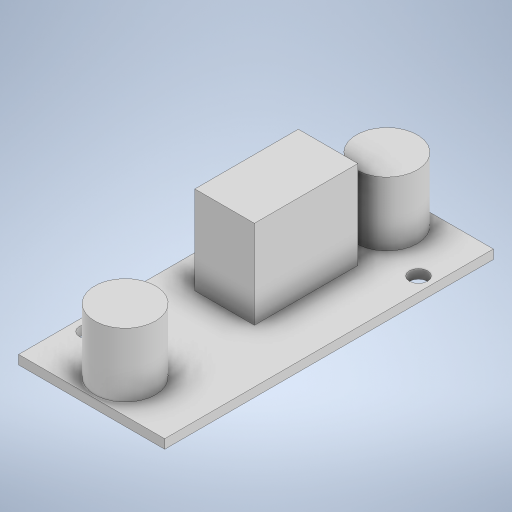
# Autodesk Inventor part: 스텝다운 컨버터
Saved by Autodesk Inventor 2023 (Build 270158000, 158)
## iProperties
Created: 2022-08-18
Part Number: 스텝다운 컨버터
Material: 일반
Document SubType Name: Modeling
Designer: user
Density: 1 g/cm^3
Appearance: 기본값
Author: user
Autodesk Inventor part; units mm, degrees
ref_plane "YZ Plane" through (0, 0, 0) normal (1, 0, 0) x (0, 1, 0)
ref_plane "XZ Plane" through (0, 0, 0) normal (0, 1, 0) x (-1, 0, 0)
ref_plane "XY Plane" through (0, 0, 0) normal (0, 0, 1) x (1, 0, 0)
sketch "스케치1" plane through (0, 0, 0) normal (0, 1, 0) x (-1, 0, 0)
  line L0 (-12, 27) -> (12, 27)
  line L1 (12, 27) -> (12, -27)
  line L2 (12, -27) -> (-12, -27)
  line L3 (-12, -27) -> (-12, 27)
  line L4 (-12, 27) -> (12, -27) construction
  line L5 (12, 27) -> (-12, -27) construction
  circle A0 centre (9.5, 18) radius 1.5
  circle A1 centre (-9.7, -17) radius 1.5
  point P0 (0, 0)
  dimension "d0" = 24
  dimension "d1" = 54
  dimension "d2" = 3
  dimension "d3" = 9
  dimension "d4" = 2.5
  dimension "d5" = 3
  dimension "d6" = 10
  dimension "d7" = 2.3
  constraints: 12 end point, 2 centre point, 2 midpoint, 2 parallel, 1 horizontal, 1 perpendicular
  measures "d0" distance of L1.end L2.end
  measures "d1" distance of L0.end L1.end
  measures "d2" diameter of A0
  measures "d3" distance from line of L0 A0.centre
  measures "d4" distance from line of L1 A0.centre
  measures "d5" diameter of A1
  measures "d6" distance from line of L2 A1.centre
  measures "d7" distance from line of L3 A1.centre
extrude "돌출1" add sketch "스케치1" along normal blind 1.5
sketch "스케치2" plane through (0, 1.5, 0) normal (0, 1, 0) x (1, 0, 0)
  circle A0 centre (0, -21.5) radius 5
  circle A1 centre (0, 21.5) radius 5
  line L0 (12, 27) -> (-12, 27) projected
  line L1 (-12, -27) -> (12, -27) projected
  point P0 (0, 0)
  dimension "d10" = 10
  dimension "d11" = 5.5
  dimension "d12" = 5.5
  dimension "d13" = 10
  constraints: 2 centre point
  measures "d10" diameter of A1
  measures "d11" distance from line of L0 A1.centre
  measures "d12" distance from line of L1 A0.centre
  measures "d13" diameter of A0
extrude "돌출2" add sketch "스케치2" along normal blind 10.5
sketch "스케치3" plane through (0, 1.5, 0) normal (0, 1, 0) x (1, 0, 0)
  line L0 (-6.5682, -3.4773) -> (3.2197, -3.4773)
  line L1 (3.2197, -3.4773) -> (3.2197, 13.5227)
  line L2 (3.2197, 13.5227) -> (-6.5682, 13.5227)
  line L3 (-6.5682, 13.5227) -> (-6.5682, -3.4773)
  line L4 (-6.5682, -3.4773) -> (3.2197, 13.5227) construction
  line L5 (3.2197, -3.4773) -> (-6.5682, 13.5227) construction
  point P0 (0, 0)
  point P1 (-1.6742, 5.0227)
  dimension "d16" = 17
  constraints: 12 end point, 2 midpoint, 2 parallel, 1 horizontal, 1 perpendicular
  measures "d16" distance of L2.end L0.start
extrude "돌출3" add sketch "스케치3" along normal blind 14.5
